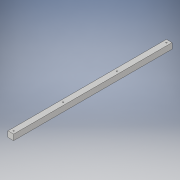
# Autodesk Inventor part: bumper runner
Saved by Autodesk Inventor 2019 (Build 230136000, 136)
## iProperties
Created: 2018-12-24
Part Number: bumper runner
Material: Generic
Document SubType Name: Modeling
Designer: Tiberus
Density: 1 g/cm^3
Appearance: Default
Author: Tiberus
Autodesk Inventor part; units mm, degrees
ref_plane "YZ Plane" through (0, 0, 0) normal (1, 0, 0) x (0, 1, 0)
ref_plane "XZ Plane" through (0, 0, 0) normal (0, 1, 0) x (-1, 0, 0)
ref_plane "XY Plane" through (0, 0, 0) normal (0, 0, 1) x (1, 0, 0)
sketch "Sketch1" plane through (0, 0, 0) normal (0, 0, 1) x (1, 0, 0)
  line L0 (0, 0) -> (25.4, 0)
  line L1 (25.4, 0) -> (25.4, 25.4)
  line L2 (25.4, 25.4) -> (0, 25.4)
  line L3 (0, 25.4) -> (0, 0)
  dimension "d0" = 25.4
  dimension "d1" = 25.4
  constraints: 8 end point, 2 parallel, 1 horizontal, 1 perpendicular
  measures "d0" distance of L2.end L1.end
  measures "d1" distance of L1.end L0.end
extrude "Extrusion1" add sketch "Sketch1" along normal blind 711.2
sketch "Sketch2" plane through (0, 25.4, 0) normal (0, 1, 0) x (1, 0, 0)
  line L0 (0, -711.2) -> (25.4, -711.2) construction
  line L1 (12.7, -711.2) -> (12.7, -698.5) construction
  circle A0 centre (12.7, -698.5) radius 2.5797
  line L2 (12.7, -711.2) -> (12.7, -476.25) construction
  circle A1 centre (12.7, -476.25) radius 2.5797
  line L3 (0, 0) -> (0, -711.2) construction
  line L4 (0, -355.6) -> (25.4, -355.6) construction
  circle A2 centre (12.7, -12.7) radius 2.5797
  circle A3 centre (12.7, -234.95) radius 2.5797
  dimension "d4" = 12.7
  dimension "d5" = 5.1594
  dimension "d6" = 234.95
  dimension "d7" = 5.1594
  constraints: 6 end point, 4 centre point, 2 coincident, 2 midpoint, 2 symmetric about line, 2 vertical, 1 horizontal, 2 other
  measures "d4" distance of L1.start L1.end
  measures "d5" diameter of A0
  measures "d6" distance of L1.start L2.end
  measures "d7" diameter of A1
extrude "Extrusion2" cut sketch "Sketch2" against normal blind 711.2
body "Solid1"
